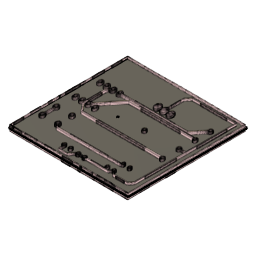
Untitled7 (Autodesk Fusion 360 design; units mm, degrees)
part number: 2026-01-31-21-15-14-512
Autodesk Fusion 360 part; units mm, degrees
sketch "Sketch1" plane through (0, 0, 0) normal (1, 0, 0) x (0, 1, 0)
sketch "Sketch2" plane through (0, 0, 0) normal (0, 0, 1) x (1, 0, 0)
  line L0 (-15, 20) -> (35.1331, 20)
  line L1 (35.1331, 20) -> (35.1331, -30)
  line L2 (35.1331, -30) -> (-15, -30)
  line L3 (-15, -30) -> (-15, 20)
  dimension "d1" = 50
  constraint horizontal L0
  constraint vertical L1
  constraint horizontal L2
  constraint vertical L3
  measures "d1" distance of L0.start L2.end
extrude "Extrude1" add sketch "Sketch2" along normal blind 0.5
other "Base Mesh Feature1"
other "Modify1"
other "Modify2"
move_body "Move1" bodies 1 to x (1, 0, 0) y (0, 1, 0) z (0, 0, 1) at (0, 0, 3)
other "Base Mesh Feature2"
other "Modify3"
other "Modify4"
other "Modify5"
other "Modify6"
other "Modify7"
move_body "Move2" bodies 1 to x (1, 0, 0) y (0, 1, 0) z (0, 0, 1) at (0, 0, -2)
other "Modify8"
sketch "Sketch3" plane through (0, 0, 1.5) normal (0, 0, 1) x (-1, 0, 0)
  line L0 (15, 30) -> (-35.1331, 30)
  line L1 (-35.1331, 30) -> (-35.1331, -20)
  line L2 (-35.1331, -20) -> (15, -20)
  line L3 (15, -20) -> (15, 30)
  circle A0 centre (6, -4.8) radius 0.3606
  circle A1 centre (3.2, -4.8) radius 0.3606
extrude "Extrude2" cut sketch "Sketch3" along normal blind 3 and the other way blind 3 contours A0 | A1
sketch "Sketch4" plane through (0, 0, 0) normal (0, 0, 1) x (1, 0, 0)
  circle A0 centre (4.1, -3.3) radius 0.4123
  circle A1 centre (-3.3, -5.5) radius 0.3606
  circle A2 centre (-6, -5.5) radius 0.4243
extrude "Extrude3" cut sketch "Sketch4" along normal blind 5 and the other way blind 2
sketch "Sketch5" plane through (0, 0, 1.5) normal (0, 0, 1) x (-1, 0, 0)
  circle A0 centre (3.3, 5.5) radius 0.3606
  circle A1 centre (6, 5.5) radius 0.4243
  circle A2 centre (-4.1, 3.3) radius 0.4123
  circle A3 centre (3.2, -4.8) radius 0.3606
  circle A4 centre (6, -4.8) radius 0.3606
  line L0 (15, 30) -> (-35.1331, 30)
  line L1 (-35.1331, 30) -> (-35.1331, -20)
  line L2 (-35.1331, -20) -> (15, -20)
  line L3 (15, -20) -> (15, 30)
  circle A5 centre (8.6909, -4.8054) radius 0.3602
  circle A6 centre (11.4199, -4.8054) radius 0.3548
extrude "Extrude4" cut sketch "Sketch5" against normal blind 3 contours A5 | A6
sketch "Sketch6" plane through (0, 0, 1.5) normal (0, 0, 1) x (-1, 0, 0)
  circle A0 centre (8.6909, -4.8054) radius 0.3602
  circle A1 centre (11.4199, -4.8054) radius 0.3548
  circle A2 centre (3.3, 5.5) radius 0.3606
  circle A3 centre (6, 5.5) radius 0.4243
  circle A4 centre (-4.1, 3.3) radius 0.4123
  circle A5 centre (3.2, -4.8) radius 0.3606
  circle A6 centre (6, -4.8) radius 0.3606
  line L0 (15, 30) -> (-35.1331, 30)
  line L1 (-35.1331, 30) -> (-35.1331, -20)
  line L2 (-35.1331, -20) -> (15, -20)
  line L3 (15, -20) -> (15, 30)
  circle A7 centre (8.6998, 5.4561) radius 0.3977
  circle A8 centre (11.3912, 5.4561) radius 0.3414
extrude "Extrude5" cut sketch "Sketch6" against normal blind 2 contours A7 | A8
sketch "Sketch7" plane through (0, 0, 1.5) normal (0, 0, 1) x (-1, 0, 0)
  circle A0 centre (8.6998, 5.4561) radius 0.3977
  circle A1 centre (11.3912, 5.4561) radius 0.3414
  circle A2 centre (8.6909, -4.8054) radius 0.3602
  circle A3 centre (11.4199, -4.8054) radius 0.3548
  circle A4 centre (3.3, 5.5) radius 0.3606
  circle A5 centre (6, 5.5) radius 0.4243
  circle A6 centre (-4.1, 3.3) radius 0.4123
  circle A7 centre (3.2, -4.8) radius 0.3606
  circle A8 centre (6, -4.8) radius 0.3606
  line L0 (15, 30) -> (-35.1331, 30)
  line L1 (-35.1331, 30) -> (-35.1331, -20)
  line L2 (-35.1331, -20) -> (15, -20)
  line L3 (15, -20) -> (15, 30)
  circle A9 centre (5.2943, 13.0782) radius 0.4402
  circle A10 centre (11.8232, 13.0782) radius 0.4821
  circle A11 centre (5.2943, 19.0796) radius 0.4177
  circle A12 centre (11.8232, 19.0796) radius 0.5294
extrude "Extrude6" cut sketch "Sketch7" against normal blind 500 contours A9 | A10 | A11 | A12
sketch "Sketch8" plane through (0, 0, 1.5) normal (0, 0, 1) x (-1, 0, 0)
  circle A0 centre (5.2943, 19.0796) radius 0.4177
  circle A1 centre (11.8232, 19.0796) radius 0.5294
  circle A2 centre (5.2943, 13.0782) radius 0.4402
  circle A3 centre (11.8232, 13.0782) radius 0.4821
  circle A4 centre (8.6998, 5.4561) radius 0.3977
  circle A5 centre (11.3912, 5.4561) radius 0.3414
  circle A6 centre (8.6909, -4.8054) radius 0.3602
  circle A7 centre (11.4199, -4.8054) radius 0.3548
  circle A8 centre (3.3, 5.5) radius 0.3606
  circle A9 centre (6, 5.5) radius 0.4243
  circle A10 centre (-4.1, 3.3) radius 0.4123
  circle A11 centre (3.2, -4.8) radius 0.3606
  circle A12 centre (6, -4.8) radius 0.3606
  line L0 (15, 30) -> (-35.1331, 30)
  line L1 (-35.1331, 30) -> (-35.1331, -20)
  line L2 (-35.1331, -20) -> (15, -20)
  line L3 (15, -20) -> (15, 30)
  circle A13 centre (-15.194, 3.303) radius 0.4306
  circle A14 centre (-29.2, 2.8) radius 0.3606
  circle A15 centre (-29.3, 9.8) radius 0.3606
  circle A16 centre (-29.4, -3.8) radius 0.4123
  circle A17 centre (-29.5, -10.2) radius 0.4243
extrude "Extrude7" cut sketch "Sketch8" against normal blind 50 contours A13 | A14 | A15 | A16 | A17
sketch "Sketch9" plane through (0, 0, 1.5) normal (0, 0, 1) x (-1, 0, 0)
  circle A0 centre (-29.2, 2.8) radius 0.3606
  circle A1 centre (-29.4, -3.8) radius 0.4123
  circle A2 centre (-29.3, 9.8) radius 0.3606
  circle A3 centre (-29.5, -10.2) radius 0.4243
  circle A4 centre (-15.194, 3.303) radius 0.4306
  circle A5 centre (5.2943, 19.0796) radius 0.4177
  circle A6 centre (11.8232, 19.0796) radius 0.5294
  circle A7 centre (5.2943, 13.0782) radius 0.4402
  circle A8 centre (11.8232, 13.0782) radius 0.4821
  circle A9 centre (8.6998, 5.4561) radius 0.3977
  circle A10 centre (11.3912, 5.4561) radius 0.3414
  circle A11 centre (8.6909, -4.8054) radius 0.3602
  circle A12 centre (11.4199, -4.8054) radius 0.3548
  circle A13 centre (3.3, 5.5) radius 0.3606
  circle A14 centre (6, 5.5) radius 0.4243
  circle A15 centre (-4.1, 3.3) radius 0.4123
  circle A16 centre (3.2, -4.8) radius 0.3606
  circle A17 centre (6, -4.8) radius 0.3606
  line L0 (15, 30) -> (-35.1331, 30)
  line L1 (-35.1331, 30) -> (-35.1331, -20)
  line L2 (-35.1331, -20) -> (15, -20)
  line L3 (15, -20) -> (15, 30)
  circle A18 centre (-23.473, 24.3607) radius 0.3314
  circle A19 centre (-20.7784, 24.3607) radius 0.3135
  circle A20 centre (-25.8292, 20.0909) radius 0.3215
  circle A21 centre (-23.1216, 20.0909) radius 0.3884
  circle A22 centre (-12.5903, 25.7275) radius 0.3072
  circle A23 centre (-9.9608, 25.7275) radius 0.3907
  circle A24 centre (-6.407, 25.389) radius 0.3437
  circle A25 centre (-3.7384, 25.389) radius 0.3319
extrude "Extrude8" cut sketch "Sketch9" against normal blind 50 contours A18 | A19 | A20 | A21 | A22 | A23 | A24 | A25
